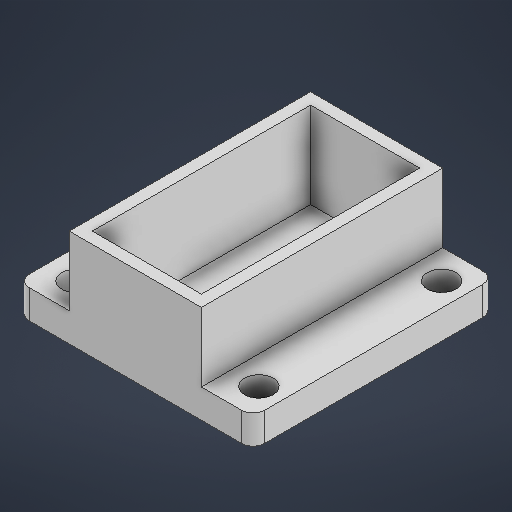
# Autodesk Inventor part: Teenscy Holder
Saved by Autodesk Inventor 2026 (Build 300175050, 175E)
## iProperties
Created: 2025-07-14
Part Number: Teenscy Holder
Material: Generic
Document SubType Name: Modeling
Designer: User
Density: 1 g/cm^3
Appearance: Default
Author: User
Autodesk Inventor part; units mm, degrees
ref_plane "YZ Plane" through (0, 0, 0) normal (1, 0, 0) x (0, 1, 0)
ref_plane "XZ Plane" through (0, 0, 0) normal (0, 1, 0) x (-1, 0, 0)
ref_plane "XY Plane" through (0, 0, 0) normal (0, 0, 1) x (1, 0, 0)
sketch "Sketch1" plane through (0, 0, 0) normal (0, 1, 0) x (-1, 0, 0)
  line L0 (19, 0) -> (0, 0)
  line L1 (0, 0) -> (0, -38)
  line L2 (0, -38) -> (19, -38)
  line L3 (19, -38) -> (19, 0)
  line L4 (21, 2) -> (-2, 2)
  line L5 (-2, 2) -> (-2, -40)
  line L6 (-2, -40) -> (21, -40)
  line L7 (21, -40) -> (21, 2)
  dimension "d0" = 19
  dimension "d1" = 38
  dimension "d2" = 90
  dimension "d3" = 90
  dimension "d9" = 42
  dimension "d10" = 2
  dimension "d11" = 2
  dimension "d12" = 2
  dimension "d30" = 22
  constraints: 16 end point, 2 horizontal, 2 perpendicular, 1 coincident, 1 parallel
  measures "d0" distance of L0.start L0.end
  measures "d1" distance of L0.end L1.end
  measures "d2" angle of L1 L0
  measures "d3" angle of L2 L3
  measures "d9" distance of L6.end L4.start
  measures "d10" distance between parallel lines of L3 L7
  measures "d11" distance between parallel lines of L6 L2
  measures "d12" horizontal distance of point (0, 0) L4.end
extrude "Extrusion1" add sketch "Sketch1" against normal blind 2 contours L3 L2 L1 L0 | L7 L6 L5 L4
sketch "Sketch2" plane through (0, 0, 0) normal (0, 1, 0) x (1, 0, 0)
  line L0 (0, 0) -> (0, 38)
  line L1 (0, 38) -> (-19, 38)
  line L2 (-19, 38) -> (-19, 0)
  line L3 (-19, 0) -> (0, 0)
  line L4 (-21, 40) -> (-21, -2) projected
  line L5 (2, 40) -> (-21, 40) projected
  line L6 (2, -2) -> (-21, -2) projected
  line L7 (-21, -2) -> (2, -2)
  line L8 (2, -2) -> (2, 40)
  line L9 (2, 40) -> (-21, 40)
  point P0 (2, 40)
  dimension "d15" = 2
  dimension "d16" = 2
  dimension "d17" = 90
  constraints: 14 end point, 4 perpendicular, 1 horizontal, 1 vertical
  measures "d15" distance between parallel lines of L4 L2
  measures "d16" distance between parallel lines of L5 L1
  measures "d17" angle of L8 L9
extrude "Extrusion2" add sketch "Sketch2" along normal blind 15
sketch "Sketch3" plane through (0, -2, 0) normal (0, -1, 0) x (1, 0, 0)
  circle A0 centre (-9, -19) radius 22.5 construction
  circle A1 centre (-24.9099, -3.0901) radius 2.5
  circle A2 centre (6.9099, -34.9099) radius 2.5
  line L0 (-24.9099, -3.0901) -> (6.9099, -34.9099) construction
  circle A3 centre (6.9099, -3.0901) radius 2.5
  line L1 (-24.9099, -34.9099) -> (6.9099, -3.0901) construction
  circle A4 centre (-24.9099, -34.9099) radius 2.5
  line L2 (-9, 3.5) -> (-9, -41.5) construction
  line L3 (2, -40) -> (2, 2) projected
  line L4 (-21, -40) -> (2, -40) projected
  line L5 (-21, 2) -> (-30, 2)
  line L6 (-30, 2) -> (-30, -40)
  line L7 (-30, -40) -> (-21, -40)
  line L8 (2, -40) -> (11, -40)
  line L9 (11, -40) -> (11, 2)
  line L10 (11, 2) -> (2, 2)
  line L11 (-21, 2) -> (-21, -40)
  point P0 (0, 0)
  point P1 (-9, -19)
  point P2 (-9, -19)
  dimension "d20" = 45
  dimension "d21" = 5
  dimension "d22" = 5
  dimension "d23" = 45
  dimension "d24" = 5
  dimension "d25" = 5
  dimension "d26" = 45
  dimension "d27" = 90
  dimension "d28" = 45
  dimension "d29" = 11
  dimension "d31" = 21
  dimension "d32" = 0
  dimension "d33" = 9
  dimension "d34" = 42
  dimension "d35" = 9
  constraints: 20 end point, 6 point on circle, 5 centre point, 3 vertical, 2 midpoint, 2 perpendicular, 1 coincident, 1 horizontal, 1 point on line
  measures "d20" diameter of A0
  measures "d21" diameter of A1
  measures "d22" diameter of A2
  measures "d23" distance of L0.start L0.end
  measures "d24" diameter of A4
  measures "d25" diameter of A3
  measures "d26" distance of L1.start L1.end
  measures "d27" angle of L0 L1
  measures "d28" angle of L2 L0
  measures "d29" distance from line of L3 point (-9, -19)
  measures "d31" distance from line of L4 point (-9, -19)
  measures "d32" distance from line of point (-9, -19) L2
  measures "d33" distance of L5.start L5.end
  measures "d34" distance of L5.end L6.end
  measures "d35" distance of L3.start L8.end
extrude "Extrusion3" add sketch "Sketch3" against normal blind 5
fillet "Fillet1" radius 2 4 edges at (11, 0.5, 2) (11, 0.5, -40) (-30, 0.5, -40) (-30, 0.5, 2)
body "Solid1"
